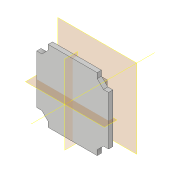
# Autodesk Inventor part: 20_Cube_Insert_Lightsheet_Flowcube_rectangular_v3
Saved by Autodesk Inventor 2022 (Build 260153000, 153)
## iProperties
Created: 2019-07-01
Part Number: 20_Cube_Insert_Lightsheet_Flowcube_rectangular_v3
Material: Generic
Document SubType Name: Modeling
Designer: diederichbenedict
Density: 1 g/cm^3
Appearance: Default
Author: diederichbenedict
Autodesk Inventor part; units mm, degrees
ref_plane "YZ Plane" through (0, 0, 0) normal (1, 0, 0) x (0, 1, 0)
ref_plane "XZ Plane" through (0, 0, 0) normal (0, 1, 0) x (-1, 0, 0)
ref_plane "Work Plane1" through (0, 0, 10) normal (0, 0, 1) x (1, 0, 0)
sketch "Sketch1" plane through (0, 0, 10) normal (0, 0, 1) x (1, 0, 0)
  line L0 (-4.0299, -0.3538) -> (-2.2322, 1.4439) construction
  arc A0 (-1.4439, 2.2322) -> (-2.2322, 1.4439) centre (-0.9299, 0.9299) ccw construction
  line L1 (-1.4439, 2.2322) -> (0.3538, 4.0299) construction
  line L2 (-37.8299, 42.8299) -> (-37.8299, 37.8299) construction
  line L3 (-37.8299, 37.8299) -> (-42.9208, 37.8299) construction
  line L4 (-37.8299, 42.2137) -> (-37.8299, 45.8299) construction
  line L5 (-37.8299, 45.8299) -> (-4.0299, 45.8299) construction
  line L6 (-4.0299, 45.8299) -> (-4.0299, 42.2137) construction
  line L7 (-4.0299, 4.0299) -> (0.3538, 4.0299) projected
  circle A1 centre (-20.9299, 20.9299) radius 17.5 projected
  line L8 (-20.9299, 58.9723) -> (17.1124, 20.9299) construction
  line L9 (17.1124, 20.9299) -> (-20.9299, -17.1124) construction
  line L10 (-20.9299, -17.1124) -> (-58.9723, 20.9299) construction
  line L11 (-58.9723, 20.9299) -> (-20.9299, 58.9723) construction
  line L12 (-20.9299, 58.9723) -> (-20.9299, -17.1124) construction
  line L13 (17.1124, 20.9299) -> (-58.9723, 20.9299) construction
  line L14 (-20.9299, 58.9723) -> (32.8701, 58.9723) construction
  line L15 (-43.4299, 43.4299) -> (1.5701, 43.4299) construction
  line L16 (1.5701, 43.4299) -> (1.5701, -1.5701) construction
  line L17 (1.5701, -1.5701) -> (-43.4299, -1.5701) construction
  line L18 (-43.4299, -1.5701) -> (-43.4299, 43.4299) construction
  line L19 (-43.4299, 43.4299) -> (1.5701, -1.5701) construction
  line L20 (1.5701, 43.4299) -> (-43.4299, -1.5701) construction
  line L21 (-43.4299, 5.3876) -> (-43.4299, 36.4723)
  line L22 (-43.4299, 36.4723) -> (-36.4723, 43.4299)
  line L23 (-36.4723, 43.4299) -> (-5.3876, 43.4299)
  line L24 (-5.3876, 43.4299) -> (1.5701, 36.4723)
  line L25 (1.5701, 36.4723) -> (1.5701, 5.3876)
  line L26 (1.5701, 5.3876) -> (-5.3876, -1.5701)
  line L27 (-5.3876, -1.5701) -> (-36.4723, -1.5701)
  line L28 (-36.4723, -1.5701) -> (-43.4299, 5.3876)
  line L29 (-4.0299, 42.2137) -> (-37.8299, 42.2137) projected
  line L30 (-4.0299, -0.3538) -> (-4.0299, 4.0299) projected
  circle A2 centre (-20.9299, 20.9299) radius 1.5
  line L31 (-10.9299, 10.9299) -> (-30.9299, 10.9299) construction
  line L32 (-30.9299, 10.9299) -> (-30.9299, 30.9299) construction
  line L33 (-30.9299, 30.9299) -> (-10.9299, 30.9299) construction
  line L34 (-10.9299, 30.9299) -> (-10.9299, 10.9299) construction
  line L35 (-10.9299, 10.9299) -> (-30.9299, 30.9299) construction
  line L36 (-30.9299, 10.9299) -> (-10.9299, 30.9299) construction
  circle A3 centre (-30.9299, 30.9299) radius 1.4
  circle A4 centre (-30.9299, 10.9299) radius 1.4
  circle A5 centre (-10.9299, 10.9299) radius 1.4
  line L37 (-45.8299, 37.8299) -> (-42.0723, 37.8299) construction
  line L38 (-42.1723, 37.7299) -> (-45.8299, 37.7299)
  line L39 (-45.8299, 37.7299) -> (-45.8299, 4.1299)
  line L40 (-45.8299, 4.1299) -> (-42.1723, 4.1299)
  line L41 (-42.1723, 4.1299) -> (-42.1723, 37.7299)
  line L42 (-45.8299, 4.0299) -> (-42.0723, 4.0299) construction
  line L43 (-45.8299, 37.8299) -> (-42.0723, 37.8299) projected
  line L44 (-37.7299, 45.8299) -> (-4.1299, 45.8299)
  line L45 (-4.1299, 45.8299) -> (-4.1299, 42.1723)
  line L46 (-4.1299, 42.1723) -> (-37.7299, 42.1723)
  line L47 (-37.7299, 42.1723) -> (-37.7299, 45.8299)
  line L48 (0.4701, 37.8299) -> (0.4701, 4.0299) construction
  line L49 (0.4701, 4.0299) -> (3.9701, 4.0299) construction
  line L50 (3.9701, 37.8299) -> (3.9701, 4.0299) construction
  line L51 (0.4701, 37.8299) -> (3.9701, 37.8299) construction
  line L52 (-45.8299, -3.9701) -> (-4.0299, -3.9701) construction
  line L53 (0.3124, 37.7299) -> (3.9701, 37.7299)
  line L54 (3.9701, 37.7299) -> (3.9701, 4.1299)
  line L55 (3.9701, 4.1299) -> (0.3124, 4.1299)
  line L56 (0.3124, 4.1299) -> (0.3124, 37.7299)
  line L57 (-4.1713, -0.3538) -> (-37.7299, -0.3538)
  line L58 (-37.7299, -0.3538) -> (-37.7299, -3.9701)
  line L59 (-37.7299, -3.9701) -> (-4.1713, -3.9701)
  line L60 (-4.1713, -3.9701) -> (-4.1713, -0.3538)
  point P0 (-37.8299, 4.0299)
  dimension "d18" = 53.8
  dimension "d19" = 45
  dimension "d20" = 53.8
  dimension "d21" = 45
  dimension "d22" = 45
  dimension "d30" = 20
  dimension "d31" = 20
  dimension "d32" = 2.8
  dimension "d33" = 2.8
  dimension "d34" = 2.8
  dimension "d35" = 3
  dimension "d36" = 0.1
  dimension "d37" = 0.1
  dimension "d38" = 0.1
  dimension "d39" = 0.1
  constraints: 86 end point, 21 point on line, 14 parallel, 8 perpendicular, 7 horizontal, 7 midpoint, 4 centre point, 4 coincident, 1 equal length
  measures "d18" distance of L8.start L8.end
  measures "d19" angle of L8 L14
  measures "d20" distance of L8.end L9.end
  measures "d21" distance of L16.end L17.end
  measures "d22" distance of L15.end L16.end
  measures "d30" distance of L32.end L33.end
  measures "d31" distance of L31.end L32.end
  measures "d32" diameter of A3
  measures "d33" diameter of A4
  measures "d34" diameter of A5
  measures "d35" diameter of A2
  measures "d36" distance between parallel lines of L38 L43
  measures "d37" distance between parallel lines of L40 L42
  measures "d38" distance between parallel lines of L45 L6
  measures "d39" distance between parallel lines of L4 L47
extrude "Extrusion1" add sketch "Sketch1" along normal blind 3 contours L30 L26 L57 L28 L41 L22 L46 L24 L56 L7 | L7 L26 L30 | L56 L24 L25 L26 | L26 L25 L24 L53 L54 L55 | L60 L59 L58 L57 L28 L27 L26 | L26 L27 L28 L57 | L46 L22 L29 L24 | L24 L29 L45 | L40 L39 L38 L22 L21 L28 | L28 L21 L22 L41 | L29 L22 L23 L24 | L24 L23 L22 L29 L47 L44 L45 | L47 L29 L22 | A1 | A2 | A3 | A4 | A5
sketch "Skizze4" plane through (0, 0, 13) normal (0, 0, 1) x (1, 0, 0)
  line L0 (-37.7299, 42.1723) -> (-42.1723, 37.7299) projected
  line L1 (-42.1723, 37.7299) -> (-45.8299, 37.7299) projected
  line L2 (-45.8299, 37.7299) -> (-45.8299, 4.1299) construction
  line L3 (-45.8299, 4.1299) -> (-42.1723, 4.1299) projected
  line L4 (-42.1723, 4.1299) -> (-37.6885, -0.3538) projected
  line L5 (-37.6885, -0.3538) -> (-37.7299, -0.3538) projected
  line L6 (-37.7299, -0.3538) -> (-37.7299, -3.9701) projected
  line L7 (-37.7299, -3.9701) -> (-4.1713, -3.9701) construction
  line L8 (-4.1713, -3.9701) -> (-4.1713, -0.3538) projected
  line L9 (-4.1713, -0.3538) -> (0.3124, 4.1299) projected
  line L10 (0.3124, 4.1299) -> (3.9701, 4.1299) projected
  line L11 (3.9701, 4.1299) -> (3.9701, 37.7299) construction
  line L12 (3.9701, 37.7299) -> (0.3124, 37.7299) projected
  line L13 (0.3124, 37.7299) -> (-4.1299, 42.1723) projected
  line L14 (-4.1299, 42.1723) -> (-4.1299, 45.8299) projected
  line L15 (-4.1299, 45.8299) -> (-37.7299, 45.8299) construction
  line L16 (-37.7299, 45.8299) -> (-37.7299, 42.1723) projected
  line L17 (-37.9299, 46.0299) -> (-3.9299, 46.0299) construction
  line L18 (-3.9299, 46.0299) -> (-3.9299, 42.2551)
  line L19 (-3.9299, 42.2551) -> (0.3953, 37.9299)
  line L20 (0.3953, 37.9299) -> (4.1701, 37.9299)
  line L21 (4.1701, 37.9299) -> (4.1701, 3.9299) construction
  line L22 (4.1701, 3.9299) -> (0.3953, 3.9299)
  line L23 (0.3953, 3.9299) -> (-3.9713, -0.4367)
  line L24 (-3.9713, -0.4367) -> (-3.9713, -4.1701)
  line L25 (-3.9713, -4.1701) -> (-37.9299, -4.1701) construction
  line L26 (-37.9299, -4.1701) -> (-37.9299, -0.3953)
  line L27 (-37.9299, -0.3953) -> (-42.2551, 3.9299)
  line L28 (-42.2551, 3.9299) -> (-46.0299, 3.9299)
  line L29 (-46.0299, 3.9299) -> (-46.0299, 37.9299) construction
  line L30 (-46.0299, 37.9299) -> (-42.2551, 37.9299)
  line L31 (-42.2551, 37.9299) -> (-37.9299, 42.2551)
  line L32 (-37.9299, 42.2551) -> (-37.9299, 46.0299)
  line L33 (-45.8299, 37.7299) -> (-45.8299, 37.9299)
  line L34 (-4.1299, 45.8299) -> (-37.7299, 45.8299) projected
  line L35 (-37.7299, 45.8299) -> (-37.9299, 45.8299)
  line L36 (-4.1299, 45.8299) -> (-3.9299, 45.8299)
  line L37 (3.9701, 37.7299) -> (3.9701, 37.9299)
  line L38 (3.9701, 4.1299) -> (3.9701, 37.7299) projected
  line L39 (3.9701, 4.1299) -> (3.9701, 3.9299)
  line L40 (-4.1713, -3.9701) -> (-3.9713, -3.9701)
  line L41 (-37.7299, -3.9701) -> (-37.9299, -3.9701)
  line L42 (-45.8299, 4.1299) -> (-45.8299, 3.9299)
  point P0 (0, 0)
  dimension "d40" = 0.2
  constraints: 48 end point, 12 point on line, 4 perpendicular, 15 other
  measures "d40" distance between parallel lines of L15 L17
extrude "IM_offset" add sketch "Skizze4" against normal up to surface (3 mm away)
ref_plane "Arbeitsebene5" through (-20.9299, 3.9299, 10) normal (1, 0, 0) x (0, 0, -1)
ref_plane "Arbeitsebene6" through (-37.9299, 20.9299, 10) normal (0, 1, 0) x (1, 0, 0)
sketch "Skizze36" plane through (0, 0, 10) normal (0, 0, -1) x (-1, 0, 0)
  line L0 (-13.9301, 20.9299) -> (55.7899, 20.9299) projected
  line L1 (20.9299, -13.9301) -> (20.9299, 55.7899) projected
  line L2 (19.9299, 21.9299) -> (39.9299, 21.9299)
  line L3 (39.9299, 21.9299) -> (39.9299, 1.9299)
  line L4 (39.9299, 1.9299) -> (19.9299, 1.9299)
  line L5 (19.9299, 1.9299) -> (19.9299, 21.9299)
  line L6 (39.9299, 1.9299) -> (27.9299, 1.9299)
  line L7 (27.9299, 1.9299) -> (27.9299, 13.9299)
  line L8 (27.9299, 13.9299) -> (39.9299, 13.9299)
  line L9 (39.9299, 13.9299) -> (39.9299, 1.9299)
  point P0 (0, 0)
  point P1 (39.9299, 13.9299)
  point P2 (39.9299, 20.9299)
  point P3 (20.9299, 20.9299)
  point P4 (20.9299, 1.9299)
  point P5 (27.9299, 1.9299)
  dimension "d197" = 20
  dimension "d198" = 20
  dimension "d199" = 1
  dimension "d200" = 1
  dimension "d201" = 12
  dimension "d202" = 12
  constraints: 16 end point, 4 parallel, 2 horizontal, 2 perpendicular
  measures "d197" distance of L3.end L4.end
  measures "d198" distance of L2.end L3.end
  measures "d199" distance between parallel lines of L2 L0
  measures "d200" distance between parallel lines of L1 L5
  measures "d201" distance of L7.end L8.end
  measures "d202" distance of L6.end L7.end
extrude "Extrusion32" add sketch "Skizze36" along normal blind 20 contours L5 L2 L1 L0 | L0 L1 L4 L5 | L1 L2 L3 L0 | L0 L3 L8 L7 L4 L1
ref_plane "Arbeitsebene10" through (0, 0, -4) normal (0, 0, 1) x (1, 0, 0)
sketch "Skizze37" plane through (0, 0, -4) normal (0, 0, 1) x (1, 0, 0)
  line L0 (-19.9299, 1.3901) -> (-19.9299, 21.9308)
  line L1 (-19.9299, 21.9308) -> (-19.9299, 13.3467)
  line L2 (-19.9299, 13.3467) -> (-21.9299, 13.3467)
  line L3 (-21.9299, 13.3467) -> (-21.9299, 17.9308)
  line L4 (-21.9299, 21.9308) -> (-19.9299, 21.9308)
  line L5 (-40.9299, 1.3901) -> (-19.9299, 1.3901)
  line L6 (-22.807, 4.3901) -> (-22.807, 7.3107)
  line L7 (-23.807, 7.3107) -> (-23.807, 4.3901)
  line L8 (-22.807, 7.3107) -> (-22.807, 9.7285) construction
  line L9 (-22.807, 9.7285) -> (-20.1457, 10.6003) construction
  line L10 (-20.1457, 10.6003) -> (-19.9299, 13.3467) construction
  spline S0 degree 3 poles (-22.807, 7.3107) (-22.807, 9.7285) (-20.1457, 10.6003) (-19.9299, 13.3467) knots 1 1 1 1 2 2 2 2
  spline S1 degree 3 poles (-23.807, 7.3107) (-23.807, 11.2353) (-23.1457, 11.6741) (-21.9299, 13.3467) knots 1 1 1 1 2 2 2 2
  line L11 (-23.807, 7.3107) -> (-23.807, 11.2353) construction
  line L12 (-23.807, 11.2353) -> (-23.1457, 11.6741) construction
  line L13 (-23.1457, 11.6741) -> (-21.9299, 13.3467) construction
  line L14 (-21.9299, 21.9308) -> (-21.9299, 19.9308)
  line L15 (-23.9299, 19.9308) -> (-28.9019, 19.9308)
  line L16 (-28.9019, 19.9308) -> (-28.9019, 21.9308)
  line L17 (-28.9019, 21.9308) -> (-21.9299, 21.9308)
  line L18 (-19.9299, 21.9308) -> (-29.9299, 11.9308) construction
  line L19 (-28.9019, 21.9308) -> (-28.9019, 19.9308)
  line L20 (-31.2605, 21.715) -> (-28.9019, 21.9308) construction
  spline S2 degree 3 poles (-34.55, 19.0538) (-32.1323, 19.0538) (-31.2605, 21.715) (-28.9019, 21.9308) knots 1 1 1 1 2 2 2 2
  line L21 (-34.55, 19.0538) -> (-32.1323, 19.0538) construction
  line L22 (-32.1323, 19.0538) -> (-31.2605, 21.715) construction
  line L23 (-30.1867, 18.715) -> (-28.9019, 19.9308) construction
  spline S3 degree 3 poles (-34.55, 18.0538) (-30.6255, 18.0538) (-30.1867, 18.715) (-28.9019, 19.9308) knots 1 1 1 1 2 2 2 2
  line L24 (-34.55, 18.0538) -> (-30.6255, 18.0538) construction
  line L25 (-30.6255, 18.0538) -> (-30.1867, 18.715) construction
  line L26 (-37.4706, 19.0538) -> (-34.55, 19.0538)
  line L27 (-34.55, 18.0538) -> (-37.4706, 18.0538)
  line L28 (-40.4706, 18.0538) -> (-40.4706, 19.0538)
  line L29 (-22.807, 4.3901) -> (-23.807, 4.3901)
  line L30 (-37.4706, 18.0538) -> (-37.4706, 19.0538)
  arc A0 (-21.9299, 17.9308) -> (-23.9299, 19.9308) centre (-23.9299, 17.9308) ccw
  line L31 (-19.9299, 1.9299) -> (-19.9299, 21.9299) projected
  point P0 (0, 0)
  point P1 (-22.807, 1.3901)
  point P2 (-40.4706, 21.9308)
  point P3 (-19.9299, 13.3467)
  dimension "d206" = 2
  dimension "d207" = 2
  dimension "d208" = 1
  dimension "d209" = 3
  dimension "d210" = 3
  dimension "d211" = 2
  dimension "d214" = 0
  constraints: 38 end point, 9 symmetric about line, 5 parallel, 3 perpendicular, 3 point on line, 2 point on circle, 2 tangent, 1 centre point, 12 other
  measures "d206" distance of L2.start L13.end
  measures "d207" distance of L15.end L17.start
  measures "d208" distance between parallel lines of L7 L6
  measures "d209" distance between parallel lines of L5 L29
  measures "d210" distance between parallel lines of L30 L28
  measures "d211" radius of A0
  measures "d214" distance between parallel lines of L31 L0
extrude "Extrusion33" cut sketch "Skizze37" along normal mid plane 2
ref_plane "Arbeitsebene11" through (-19.9299, 21.9299, 10) normal (0.7071, -0.7071, 0) x (0, 0, -1)
sketch "Skizze38" plane through (-39.9299, 13.9299, 10) normal (-1, 0, 0) x (0, 0, 1)
  line L0 (-13, 8) -> (-15, 8) projected
  line L1 (-15, 4.1239) -> (-13, 4.1239) projected
  line L2 (-15, 5.1239) -> (-13, 5.1239) projected
  circle A0 centre (-13, 4.6008) radius 0.75
  point P0 (-10, -13.9299)
  dimension "d215" = 1.5
  constraints: 1 centre point
  measures "d215" diameter of A0
extrude "Extrusion34" cut sketch "Skizze38" against normal blind 5
mirror "Spiegeln3" about plane through (-19.9299, 21.9299, 10) normal (0.7071, -0.7071, 0) of "Extrusion34"
sketch "Skizze39" plane through (0, 0, -3) normal (0, 0, -1) x (-1, 0, 0)
  line L0 (39.9299, 13.9299) -> (39.9299, 21.9299) projected
  line L1 (39.9299, 21.9299) -> (19.9299, 21.9299) projected
  line L2 (19.9299, 21.9299) -> (19.9299, 1.9299) projected
  line L3 (19.9299, 1.9299) -> (27.9299, 1.9299) projected
  line L4 (27.9299, 1.9299) -> (27.9299, 13.9299) projected
  line L5 (27.9299, 13.9299) -> (39.9299, 13.9299) projected
  line L6 (19.9299, 21.9299) -> (20.4299, 21.9299)
  line L7 (20.4299, 21.9299) -> (20.4299, 21.4299)
  line L8 (20.4299, 21.4299) -> (19.9299, 21.4299)
  line L9 (19.9299, 21.4299) -> (19.9299, 21.9299)
  point P0 (0, 0)
  dimension "d218" = 0.5
  dimension "d219" = 0.5
  constraints: 8 end point, 2 parallel, 1 horizontal, 1 perpendicular
  measures "d218" distance of L7.end L8.end
  measures "d219" distance of L6.end L7.end
extrude "Extrusion35" add sketch "Skizze39" along normal up to surface (2 mm away) contours L7 L8 L2 L1
body "Solid1"
